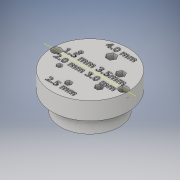
# Autodesk Inventor part: AllenKeyHolder
Saved by Autodesk Inventor 2019.1 (Build 231200000, 200)
## iProperties
Created: 2018-08-31
Part Number: AllenKeyHolder
Material: Generic
Document SubType Name: Modeling
Designer: steele
Density: 1 g/cm^3
Appearance: Default
Author: steele
Autodesk Inventor part; units mm, degrees
(part 1 of 2)
ref_plane "YZ Plane" through (0, 0, 0) normal (1, 0, 0) x (0, 1, 0)
ref_plane "XZ Plane" through (0, 0, 0) normal (0, 1, 0) x (-1, 0, 0)
ref_plane "XY Plane" through (0, 0, 0) normal (0, 0, 1) x (1, 0, 0)
sketch "Sketch1" plane through (0, 0, 0) normal (0, 1, 0) x (-1, 0, 0)
  circle A0 centre (0, 0) radius 20.574
  dimension "d0" = 41.148
  constraints: 1 centre point, 1 coincident
  measures "d0" diameter of A0
extrude "Extrusion1" add sketch "Sketch1" against normal blind 9.525
sketch "Sketch2" plane through (0, -9.525, 0) normal (0, -1, 0) x (1, 0, 0)
  circle A0 centre (0, 0) radius 15.875
  dimension "d3" = 31.75
  constraints: 1 centre point, 1 coincident
  measures "d3" diameter of A0
extrude "Extrusion2" add sketch "Sketch2" along normal blind 9.525
sketch "Sketch4" plane through (0, 0, 0) normal (0, 1, 0) x (1, 0, 0)
  circle A0 centre (0, 0) radius 20.574 projected
  point P0 (18.2245, 0)
  point P1 (-18.2245, 0)
  dimension "d9" = 18.2245
  dimension "d10" = 18.2245
  measures "d9" distance of point (18.224, 0) A0.centre
  measures "d10" distance of point (0, 0) point (-18.224, 0)
hole "Hole1" at (18.2245, 0, 0) at (-18.2245, 0, 0) direction (0, -1, 0) diameter 3.2766 end through all counterbore diameter 4.6482 counterbore depth 2.8448 clearance for "Socket Head Cap Screw" size "#4" standard "Ansi Unified Screw Threads"
sketch "Sketch5" plane through (0, 0, 0) normal (0, 1, 0) x (1, 0, 0)
  circle A0 centre (0, 0) radius 12.065 construction
  line L0 (2.2282, 12.0593) -> (0.9291, 9.8093)
  line L1 (0.9291, 9.8093) -> (-1.6689, 9.8093)
  line L2 (-1.6689, 9.8093) -> (-2.968, 12.0593)
  line L3 (-2.968, 12.0593) -> (-1.6689, 14.3093)
  line L4 (-1.6689, 14.3093) -> (0.9291, 14.3093)
  line L5 (0.9291, 14.3093) -> (2.2282, 12.0593)
  line L6 (12.5681, 6.35) -> (11.4134, 4.35)
  line L7 (11.4134, 4.35) -> (9.104, 4.35)
  line L8 (9.104, 4.35) -> (7.9493, 6.35)
  line L9 (7.9493, 6.35) -> (9.104, 8.35)
  line L10 (9.104, 8.35) -> (11.4134, 8.35)
  line L11 (11.4134, 8.35) -> (12.5681, 6.35)
  line L12 (-28.8036, 0) -> (28.8036, 0) projected
  line L13 (11.639, -3.9593) -> (12.6494, -5.7093)
  line L14 (12.6494, -5.7093) -> (11.639, -7.4593)
  line L15 (11.639, -7.4593) -> (9.6183, -7.4593)
  line L16 (9.6183, -7.4593) -> (8.6079, -5.7093)
  line L17 (8.6079, -5.7093) -> (9.6183, -3.9593)
  line L18 (9.6183, -3.9593) -> (11.639, -3.9593)
  line L19 (1.2359, -10.5593) -> (2.1019, -12.0593)
  line L20 (2.1019, -12.0593) -> (1.2359, -13.5593)
  line L21 (1.2359, -13.5593) -> (-0.4961, -13.5593)
  line L22 (-0.4961, -13.5593) -> (-1.3622, -12.0593)
  line L23 (-1.3622, -12.0593) -> (-0.4961, -10.5593)
  line L24 (-0.4961, -10.5593) -> (1.2359, -10.5593)
  line L25 (-8.8154, -6.35) -> (-9.5371, -7.6)
  line L26 (-9.5371, -7.6) -> (-10.9804, -7.6)
  line L27 (-10.9804, -7.6) -> (-11.7021, -6.35)
  line L28 (-11.7021, -6.35) -> (-10.9804, -5.1)
  line L29 (-10.9804, -5.1) -> (-9.5371, -5.1)
  line L30 (-9.5371, -5.1) -> (-8.8154, -6.35)
  line L31 (-9.4739, 5.7093) -> (-10.0513, 4.7093)
  line L32 (-10.0513, 4.7093) -> (-11.206, 4.7093)
  line L33 (-11.206, 4.7093) -> (-11.7833, 5.7093)
  line L34 (-11.7833, 5.7093) -> (-11.206, 6.7093)
  line L35 (-11.206, 6.7093) -> (-10.0513, 6.7093)
  line L36 (-10.0513, 6.7093) -> (-9.4739, 5.7093)
  point P0 (-0.3699, 12.0593)
  point P1 (-10.6286, 5.7093)
  point P2 (-10.2587, -6.35)
  point P3 (0.3699, -12.0593)
  point P4 (10.6286, -5.7093)
  point P5 (10.2587, 6.35)
  point P6 (-0.3699, 12.0593)
  point P7 (10.2587, 6.35)
  point P8 (10.6286, -5.7093)
  point P9 (0.3699, -12.0593)
  point P10 (-10.2587, -6.35)
  point P11 (-10.6286, 5.7093)
  dimension "d18" = 24.13
  dimension "d21" = 360
  dimension "d23" = 4.5
  dimension "d24" = 4
  dimension "d25" = 3.5
  dimension "d26" = 3
  dimension "d27" = 2.5
  dimension "d28" = 2
  constraints: 72 end point, 7 coincident, 5 parallel, 88 other
  measures "d23" distance between parallel lines of L1 L4
  measures "d24" distance between parallel lines of L7 L10
  measures "d25" distance between parallel lines of L15 L18
  measures "d26" distance between parallel lines of L21 L24
  measures "d27" distance between parallel lines of L26 L29
  measures "d28" distance between parallel lines of L32 L35
extrude "Extrusion4" cut sketch "Sketch5" against normal through all
sketch "Sketch6" plane through (0, 0, 0) normal (0, 1, 0) x (1, 0, 0)
  line L0 (-12.7271, 15.24) -> (13.8214, 15.24) construction
  circle A0 centre (0, 0) radius 20.574 construction
  line L1 (-11.7818, -16.8665) -> (11.7818, -16.8665) construction
  line L2 (-20.5348, 1.27) -> (20.5348, 1.27) construction
  line L3 (-20.1938, -3.937) -> (20.1938, -3.937) construction
  line L4 (-4.8017, 15.9514) -> (-5.2142, 15.9514)
  line L5 (-5.2142, 15.9514) -> (-5.2142, 15.2326)
  line L6 (-5.2142, 15.2326) -> (-5.9527, 15.2326)
  line L7 (-5.9527, 15.2326) -> (-5.9527, 15.9514)
  line L8 (-5.9527, 15.9514) -> (-7.2964, 15.9514)
  line L9 (-7.2964, 15.9514) -> (-7.2964, 16.5195)
  line L10 (-7.2964, 16.5195) -> (-5.9774, 18.288)
  line L11 (-5.9774, 18.288) -> (-5.2142, 18.288)
  line L12 (-5.2142, 18.288) -> (-5.2142, 16.4997)
  line L13 (-5.2142, 16.4997) -> (-4.8017, 16.4997)
  line L14 (-4.8017, 16.4997) -> (-4.8017, 15.9514)
  line L15 (-5.9527, 16.4997) -> (-5.9527, 17.5371)
  line L16 (-5.9527, 17.5371) -> (-6.7258, 16.4997)
  line L17 (-6.7258, 16.4997) -> (-5.9527, 16.4997)
  line L18 (-3.7025, 15.24) -> (-4.4262, 15.24)
  line L19 (-4.4262, 15.24) -> (-4.4262, 16.0452)
  line L20 (-4.4262, 16.0452) -> (-3.7025, 16.0452)
  line L21 (-3.7025, 16.0452) -> (-3.7025, 15.24)
  spline S0 degree 2 poles (-0.899, 16.764) (-0.899, 16.3688) (-1.025, 15.776) (-1.1658, 15.5759) knots 0 0 0 1 2 2 2
  spline S1 degree 2 poles (-1.1658, 15.5759) (-1.3041, 15.3783) (-1.7512, 15.1758) (-2.0723, 15.1758) knots 0 0 0 1 2 2 2
  spline S2 degree 2 poles (-2.0723, 15.1758) (-2.3959, 15.1758) (-2.8405, 15.3783) (-2.9813, 15.5809) knots 0 0 0 1 2 2 2
  spline S3 degree 2 poles (-2.9813, 15.5809) (-3.1221, 15.7809) (-3.248, 16.3688) (-3.248, 16.764) knots 0 0 0 1 2 2 2
  spline S4 degree 2 poles (-3.248, 16.764) (-3.248, 17.1691) (-3.1221, 17.7421) (-2.9788, 17.9496) knots 0 0 0 1 2 2 2
  spline S5 degree 2 poles (-2.9788, 17.9496) (-2.8355, 18.1521) (-2.3835, 18.3498) (-2.0723, 18.3498) knots 0 0 0 1 2 2 2
  spline S6 degree 2 poles (-2.0723, 18.3498) (-1.7438, 18.3498) (-1.3041, 18.1423) (-1.1633, 17.9373) knots 0 0 0 1 2 2 2
  spline S7 degree 2 poles (-1.1633, 17.9373) (-1.025, 17.7372) (-0.899, 17.1469) (-0.899, 16.764) knots 0 0 0 1 2 2 2
  spline S8 degree 2 poles (-1.6672, 16.764) (-1.6672, 17.3296) (-1.8525, 17.7866) (-2.0723, 17.7866) knots 0 0 0 1 2 2 2
  spline S9 degree 2 poles (-2.0723, 17.7866) (-2.2921, 17.7866) (-2.4798, 17.3296) (-2.4798, 16.7615) knots 0 0 0 1 2 2 2
  spline S10 degree 2 poles (-2.4798, 16.7615) (-2.4798, 16.2033) (-2.2921, 15.7389) (-2.0723, 15.7389) knots 0 0 0 1 2 2 2
  spline S11 degree 2 poles (-2.0723, 15.7389) (-1.8549, 15.7389) (-1.6672, 16.2033) (-1.6672, 16.764) knots 0 0 0 1 2 2 2
  line L22 (3.5075, 15.24) -> (3.5075, 16.3886)
  spline S12 degree 2 poles (3.5075, 16.3886) (3.5075, 16.559) (3.4951, 16.7912) (3.4655, 16.8653) knots 0 0 0 1 2 2 2
  spline S13 degree 2 poles (3.4655, 16.8653) (3.4334, 16.9394) (3.3049, 17.0061) (3.1888, 17.0061) knots 0 0 0 1 2 2 2
  spline S14 degree 2 poles (3.1888, 17.0061) (3.1073, 17.0061) (2.9492, 16.9344) (2.8554, 16.8677) knots 0 0 0 1 2 2 2
  line L23 (2.8554, 16.8677) -> (2.8554, 15.24)
  line L24 (2.8554, 15.24) -> (2.1341, 15.24)
  line L25 (2.1341, 15.24) -> (2.1341, 16.3886)
  spline S15 degree 2 poles (2.1341, 16.3886) (2.1341, 16.5565) (2.1193, 16.7912) (2.0897, 16.8653) knots 0 0 0 1 2 2 2
  spline S16 degree 2 poles (2.0897, 16.8653) (2.0576, 16.9394) (1.9291, 17.0061) (1.813, 17.0061) knots 0 0 0 1 2 2 2
  spline S17 degree 2 poles (1.813, 17.0061) (1.7266, 17.0061) (1.5562, 16.9246) (1.4771, 16.8677) knots 0 0 0 1 2 2 2
  line L26 (1.4771, 16.8677) -> (1.4771, 15.24)
  line L27 (1.4771, 15.24) -> (0.7608, 15.24)
  line L28 (0.7608, 15.24) -> (0.7608, 17.5396)
  line L29 (0.7608, 17.5396) -> (1.4771, 17.5396)
  line L30 (1.4771, 17.5396) -> (1.4771, 17.2852)
  spline S18 degree 2 poles (1.4771, 17.2852) (1.6525, 17.4334) (1.9662, 17.6013) (2.1613, 17.6013) knots 0 0 0 1 2 2 2
  spline S19 degree 2 poles (2.1613, 17.6013) (2.3713, 17.6013) (2.6924, 17.4013) (2.7763, 17.2012) knots 0 0 0 1 2 2 2
  spline S20 degree 2 poles (2.7763, 17.2012) (2.9814, 17.3939) (3.3469, 17.6013) (3.5346, 17.6013) knots 0 0 0 1 2 2 2
  spline S21 degree 2 poles (3.5346, 17.6013) (3.6952, 17.6013) (3.9496, 17.5001) (4.0361, 17.3963) knots 0 0 0 1 2 2 2
  spline S22 degree 2 poles (4.0361, 17.3963) (4.1324, 17.2852) (4.2287, 16.9814) (4.2287, 16.7368) knots 0 0 0 1 2 2 2
  line L31 (4.2287, 16.7368) -> (4.2287, 15.24)
  line L32 (4.2287, 15.24) -> (3.5075, 15.24)
  line L33 (7.504, 15.24) -> (7.504, 16.3886)
  spline S23 degree 2 poles (7.504, 16.3886) (7.504, 16.559) (7.4916, 16.7912) (7.462, 16.8653) knots 0 0 0 1 2 2 2
  spline S24 degree 2 poles (7.462, 16.8653) (7.4299, 16.9394) (7.3014, 17.0061) (7.1853, 17.0061) knots 0 0 0 1 2 2 2
  spline S25 degree 2 poles (7.1853, 17.0061) (7.1038, 17.0061) (6.9457, 16.9344) (6.8519, 16.8677) knots 0 0 0 1 2 2 2
  line L34 (6.8519, 16.8677) -> (6.8519, 15.24)
  line L35 (6.8519, 15.24) -> (6.1306, 15.24)
  line L36 (6.1306, 15.24) -> (6.1306, 16.3886)
  spline S26 degree 2 poles (6.1306, 16.3886) (6.1306, 16.5565) (6.1158, 16.7912) (6.0862, 16.8653) knots 0 0 0 1 2 2 2
  spline S27 degree 2 poles (6.0862, 16.8653) (6.0541, 16.9394) (5.9256, 17.0061) (5.8095, 17.0061) knots 0 0 0 1 2 2 2
  spline S28 degree 2 poles (5.8095, 17.0061) (5.7231, 17.0061) (5.5526, 16.9246) (5.4736, 16.8677) knots 0 0 0 1 2 2 2
  line L37 (5.4736, 16.8677) -> (5.4736, 15.24)
  line L38 (5.4736, 15.24) -> (4.7573, 15.24)
  line L39 (4.7573, 15.24) -> (4.7573, 17.5396)
  line L40 (4.7573, 17.5396) -> (5.4736, 17.5396)
  line L41 (5.4736, 17.5396) -> (5.4736, 17.2852)
  spline S29 degree 2 poles (5.4736, 17.2852) (5.649, 17.4334) (5.9627, 17.6013) (6.1578, 17.6013) knots 0 0 0 1 2 2 2
  spline S30 degree 2 poles (6.1578, 17.6013) (6.3678, 17.6013) (6.6889, 17.4013) (6.7728, 17.2012) knots 0 0 0 1 2 2 2
  spline S31 degree 2 poles (6.7728, 17.2012) (6.9778, 17.3939) (7.3434, 17.6013) (7.5311, 17.6013) knots 0 0 0 1 2 2 2
  spline S32 degree 2 poles (7.5311, 17.6013) (7.6917, 17.6013) (7.9461, 17.5001) (8.0325, 17.3963) knots 0 0 0 1 2 2 2
  spline S33 degree 2 poles (8.0325, 17.3963) (8.1289, 17.2852) (8.2252, 16.9814) (8.2252, 16.7368) knots 0 0 0 1 2 2 2
  line L42 (8.2252, 16.7368) -> (8.2252, 15.24)
  line L43 (8.2252, 15.24) -> (7.504, 15.24)
  line L44 (-14.0173, 1.27) -> (-16.1143, 1.27)
  line L45 (-16.1143, 1.27) -> (-16.1143, 1.8232)
  line L46 (-16.1143, 1.8232) -> (-15.4453, 1.8232)
  line L47 (-15.4453, 1.8232) -> (-15.4453, 3.5033)
  line L48 (-15.4453, 3.5033) -> (-16.1143, 3.5033)
  line L49 (-16.1143, 3.5033) -> (-16.1143, 4.0205)
  spline S34 degree 2 poles (-16.1143, 4.0205) (-15.9676, 4.0205) (-15.6769, 4.0591) (-15.5894, 4.1002) knots 0 0 0 1 2 2 2
  spline S35 degree 2 poles (-15.5894, 4.1002) (-15.4891, 4.1517) (-15.3759, 4.3241) (-15.3656, 4.4527) knots 0 0 0 1 2 2 2
  line L50 (-15.3656, 4.4527) -> (-14.6709, 4.4527)
  line L51 (-14.6709, 4.4527) -> (-14.6709, 1.8232)
  line L52 (-14.6709, 1.8232) -> (-14.0173, 1.8232)
  line L53 (-14.0173, 1.8232) -> (-14.0173, 1.27)
  line L54 (-12.6923, 1.27) -> (-13.4462, 1.27)
  line L55 (-13.4462, 1.27) -> (-13.4462, 2.1088)
  line L56 (-13.4462, 2.1088) -> (-12.6923, 2.1088)
  line L57 (-12.6923, 2.1088) -> (-12.6923, 1.27)
  spline S36 degree 2 poles (-9.8029, 2.3455) (-9.8029, 2.0959) (-9.9727, 1.674) (-10.1399, 1.5221) knots 0 0 0 1 2 2 2
  spline S37 degree 2 poles (-10.1399, 1.5221) (-10.3072, 1.3703) (-10.7652, 1.2031) (-11.0996, 1.2031) knots 0 0 0 1 2 2 2
  spline S38 degree 2 poles (-11.0996, 1.2031) (-11.4547, 1.2057) (-11.9641, 1.3215) (-12.1314, 1.3961) knots 0 0 0 1 2 2 2
  line L58 (-12.1314, 1.3961) -> (-12.1314, 2.0882)
  line L59 (-12.1314, 2.0882) -> (-12.0593, 2.0882)
  spline S39 degree 2 poles (-12.0593, 2.0882) (-11.9976, 2.0547) (-11.8484, 1.9673) (-11.7274, 1.921) knots 0 0 0 1 2 2 2
  spline S40 degree 2 poles (-11.7274, 1.921) (-11.6142, 1.8772) (-11.3801, 1.818) (-11.2386, 1.818) knots 0 0 0 1 2 2 2
  spline S41 degree 2 poles (-11.2386, 1.818) (-11.1151, 1.818) (-10.8269, 1.8798) (-10.7394, 1.9621) knots 0 0 0 1 2 2 2
  spline S42 degree 2 poles (-10.7394, 1.9621) (-10.6751, 2.0264) (-10.6031, 2.1834) (-10.6031, 2.3146) knots 0 0 0 1 2 2 2
  spline S43 degree 2 poles (-10.6031, 2.3146) (-10.6031, 2.4278) (-10.6957, 2.5873) (-10.7703, 2.6362) knots 0 0 0 1 2 2 2
  spline S44 degree 2 poles (-10.7703, 2.6362) (-10.8784, 2.7083) (-11.1871, 2.7494) (-11.2978, 2.7494) knots 0 0 0 1 2 2 2
  spline S45 degree 2 poles (-11.2978, 2.7494) (-11.4727, 2.7494) (-11.8046, 2.6928) (-11.9255, 2.662) knots 0 0 0 1 2 2 2
  line L60 (-11.9255, 2.662) -> (-11.995, 2.662)
  line L61 (-11.995, 2.662) -> (-11.995, 4.445)
  line L62 (-11.995, 4.445) -> (-9.8904, 4.445)
  line L63 (-9.8904, 4.445) -> (-9.8904, 3.8455)
  line L64 (-9.8904, 3.8455) -> (-11.2411, 3.8455)
  line L65 (-11.2411, 3.8455) -> (-11.2411, 3.3181)
  spline S46 degree 2 poles (-11.2411, 3.3181) (-11.1768, 3.3232) (-10.9993, 3.3283) (-10.9504, 3.3283) knots 0 0 0 1 2 2 2
  spline S47 degree 2 poles (-10.9504, 3.3283) (-10.7214, 3.3283) (-10.3355, 3.2357) (-10.1837, 3.1405) knots 0 0 0 1 2 2 2
  spline S48 degree 2 poles (-10.1837, 3.1405) (-10.0036, 3.0222) (-9.8029, 2.6285) (-9.8029, 2.3455) knots 0 0 0 1 2 2 2
  line L66 (-5.1819, 1.27) -> (-5.1819, 2.4664)
  spline S49 degree 2 poles (-5.1819, 2.4664) (-5.1819, 2.6439) (-5.1948, 2.8858) (-5.2256, 2.963) knots 0 0 0 1 2 2 2
  spline S50 degree 2 poles (-5.2256, 2.963) (-5.2591, 3.0402) (-5.3929, 3.1096) (-5.5138, 3.1096) knots 0 0 0 1 2 2 2
  spline S51 degree 2 poles (-5.5138, 3.1096) (-5.5987, 3.1096) (-5.7634, 3.035) (-5.8611, 2.9656) knots 0 0 0 1 2 2 2
  line L67 (-5.8611, 2.9656) -> (-5.8611, 1.27)
  line L68 (-5.8611, 1.27) -> (-6.6124, 1.27)
  line L69 (-6.6124, 1.27) -> (-6.6124, 2.4664)
  spline S52 degree 2 poles (-6.6124, 2.4664) (-6.6124, 2.6414) (-6.6279, 2.8858) (-6.6588, 2.963) knots 0 0 0 1 2 2 2
  spline S53 degree 2 poles (-6.6588, 2.963) (-6.6922, 3.0402) (-6.826, 3.1096) (-6.9469, 3.1096) knots 0 0 0 1 2 2 2
  spline S54 degree 2 poles (-6.9469, 3.1096) (-7.037, 3.1096) (-7.2145, 3.0247) (-7.2968, 2.9656) knots 0 0 0 1 2 2 2
  line L70 (-7.2968, 2.9656) -> (-7.2968, 1.27)
  line L71 (-7.2968, 1.27) -> (-8.043, 1.27)
  line L72 (-8.043, 1.27) -> (-8.043, 3.6654)
  line L73 (-8.043, 3.6654) -> (-7.2968, 3.6654)
  line L74 (-7.2968, 3.6654) -> (-7.2968, 3.4004)
  spline S55 degree 2 poles (-7.2968, 3.4004) (-7.1142, 3.5548) (-6.7874, 3.7297) (-6.5841, 3.7297) knots 0 0 0 1 2 2 2
  spline S56 degree 2 poles (-6.5841, 3.7297) (-6.3654, 3.7297) (-6.031, 3.5213) (-5.9435, 3.3129) knots 0 0 0 1 2 2 2
  spline S57 degree 2 poles (-5.9435, 3.3129) (-5.7299, 3.5136) (-5.3491, 3.7297) (-5.1536, 3.7297) knots 0 0 0 1 2 2 2
  spline S58 degree 2 poles (-5.1536, 3.7297) (-4.9863, 3.7297) (-4.7213, 3.6242) (-4.6313, 3.5162) knots 0 0 0 1 2 2 2
  spline S59 degree 2 poles (-4.6313, 3.5162) (-4.5309, 3.4004) (-4.4306, 3.0839) (-4.4306, 2.8292) knots 0 0 0 1 2 2 2
  line L75 (-4.4306, 2.8292) -> (-4.4306, 1.27)
  line L76 (-4.4306, 1.27) -> (-5.1819, 1.27)
  line L77 (-1.0189, 1.27) -> (-1.0189, 2.4664)
  spline S60 degree 2 poles (-1.0189, 2.4664) (-1.0189, 2.6439) (-1.0317, 2.8858) (-1.0626, 2.963) knots 0 0 0 1 2 2 2
  spline S61 degree 2 poles (-1.0626, 2.963) (-1.0961, 3.0402) (-1.2299, 3.1096) (-1.3508, 3.1096) knots 0 0 0 1 2 2 2
  spline S62 degree 2 poles (-1.3508, 3.1096) (-1.4357, 3.1096) (-1.6004, 3.035) (-1.6981, 2.9656) knots 0 0 0 1 2 2 2
  line L78 (-1.6981, 2.9656) -> (-1.6981, 1.27)
  line L79 (-1.6981, 1.27) -> (-2.4494, 1.27)
  line L80 (-2.4494, 1.27) -> (-2.4494, 2.4664)
  spline S63 degree 2 poles (-2.4494, 2.4664) (-2.4494, 2.6414) (-2.4649, 2.8858) (-2.4957, 2.963) knots 0 0 0 1 2 2 2
  spline S64 degree 2 poles (-2.4957, 2.963) (-2.5292, 3.0402) (-2.663, 3.1096) (-2.7839, 3.1096) knots 0 0 0 1 2 2 2
  spline S65 degree 2 poles (-2.7839, 3.1096) (-2.874, 3.1096) (-3.0515, 3.0247) (-3.1338, 2.9656) knots 0 0 0 1 2 2 2
  line L81 (-3.1338, 2.9656) -> (-3.1338, 1.27)
  line L82 (-3.1338, 1.27) -> (-3.88, 1.27)
  line L83 (-3.88, 1.27) -> (-3.88, 3.6654)
  line L84 (-3.88, 3.6654) -> (-3.1338, 3.6654)
  line L85 (-3.1338, 3.6654) -> (-3.1338, 3.4004)
  spline S66 degree 2 poles (-3.1338, 3.4004) (-2.9512, 3.5548) (-2.6244, 3.7297) (-2.4211, 3.7297) knots 0 0 0 1 2 2 2
  spline S67 degree 2 poles (-2.4211, 3.7297) (-2.2024, 3.7297) (-1.868, 3.5213) (-1.7805, 3.3129) knots 0 0 0 1 2 2 2
  spline S68 degree 2 poles (-1.7805, 3.3129) (-1.5669, 3.5136) (-1.1861, 3.7297) (-0.9906, 3.7297) knots 0 0 0 1 2 2 2
  spline S69 degree 2 poles (-0.9906, 3.7297) (-0.8233, 3.7297) (-0.5583, 3.6242) (-0.4683, 3.5162) knots 0 0 0 1 2 2 2
  spline S70 degree 2 poles (-0.4683, 3.5162) (-0.3679, 3.4004) (-0.2676, 3.0839) (-0.2676, 2.8292) knots 0 0 0 1 2 2 2
  line L86 (-0.2676, 2.8292) -> (-0.2676, 1.27)
  line L87 (-0.2676, 1.27) -> (-1.0189, 1.27)
  spline S71 degree 2 poles (3.8543, 2.2323) (3.8543, 1.9981) (3.6819, 1.6148) (3.5146, 1.481) knots 0 0 0 1 2 2 2
  spline S72 degree 2 poles (3.5146, 1.481) (3.3474, 1.3472) (2.892, 1.2031) (2.5652, 1.2031) knots 0 0 0 1 2 2 2
  spline S73 degree 2 poles (2.5652, 1.2031) (2.1947, 1.2031) (1.6647, 1.3266) (1.4974, 1.4038) knots 0 0 0 1 2 2 2
  line L88 (1.4974, 1.4038) -> (1.4974, 2.0933)
  line L89 (1.4974, 2.0933) -> (1.5746, 2.0933)
  spline S74 degree 2 poles (1.5746, 2.0933) (1.7496, 1.9827) (2.2204, 1.818) (2.416, 1.818) knots 0 0 0 1 2 2 2
  spline S75 degree 2 poles (2.416, 1.818) (2.5318, 1.818) (2.8019, 1.8592) (2.8945, 1.9261) knots 0 0 0 1 2 2 2
  spline S76 degree 2 poles (2.8945, 1.9261) (2.9666, 1.9801) (3.0541, 2.1371) (3.0541, 2.2786) knots 0 0 0 1 2 2 2
  spline S77 degree 2 poles (3.0541, 2.2786) (3.0541, 2.4201) (2.9306, 2.5719) (2.8277, 2.6079) knots 0 0 0 1 2 2 2
  spline S78 degree 2 poles (2.8277, 2.6079) (2.7247, 2.6439) (2.4391, 2.6517) (2.3285, 2.6517) knots 0 0 0 1 2 2 2
  line L90 (2.3285, 2.6517) -> (2.1921, 2.6517)
  line L91 (2.1921, 2.6517) -> (2.1921, 3.21)
  line L92 (2.1921, 3.21) -> (2.3182, 3.21)
  spline S79 degree 2 poles (2.3182, 3.21) (2.4623, 3.21) (2.7067, 3.2357) (2.7916, 3.2743) knots 0 0 0 1 2 2 2
  spline S80 degree 2 poles (2.7916, 3.2743) (2.8765, 3.3155) (2.9717, 3.4596) (2.9717, 3.5831) knots 0 0 0 1 2 2 2
  spline S81 degree 2 poles (2.9717, 3.5831) (2.9717, 3.6808) (2.8817, 3.8018) (2.8174, 3.8352) knots 0 0 0 1 2 2 2
  spline S82 degree 2 poles (2.8174, 3.8352) (2.7402, 3.8738) (2.5343, 3.8995) (2.4623, 3.8995) knots 0 0 0 1 2 2 2
  spline S83 degree 2 poles (2.4623, 3.8995) (2.3465, 3.8995) (2.1021, 3.8455) (1.9889, 3.8018) knots 0 0 0 1 2 2 2
  spline S84 degree 2 poles (1.9889, 3.8018) (1.8988, 3.7683) (1.7033, 3.6603) (1.657, 3.632) knots 0 0 0 1 2 2 2
  line L93 (1.657, 3.632) -> (1.5901, 3.632)
  line L94 (1.5901, 3.632) -> (1.5901, 4.3112)
  spline S85 degree 2 poles (1.5901, 4.3112) (1.7547, 4.3807) (2.3105, 4.5119) (2.6012, 4.5119) knots 0 0 0 1 2 2 2
  spline S86 degree 2 poles (2.6012, 4.5119) (2.8843, 4.5119) (3.3011, 4.4141) (3.4477, 4.3189) knots 0 0 0 1 2 2 2
  spline S87 degree 2 poles (3.4477, 4.3189) (3.6098, 4.2186) (3.7719, 3.9098) (3.7719, 3.7169) knots 0 0 0 1 2 2 2
  spline S88 degree 2 poles (3.7719, 3.7169) (3.7719, 3.4441) (3.458, 3.0376) (3.2007, 2.9784) knots 0 0 0 1 2 2 2
  line L95 (3.2007, 2.9784) -> (3.2007, 2.9476)
  spline S89 degree 2 poles (3.2007, 2.9476) (3.3139, 2.9321) (3.5301, 2.8498) (3.633, 2.7572) knots 0 0 0 1 2 2 2
  spline S90 degree 2 poles (3.633, 2.7572) (3.7282, 2.6748) (3.8543, 2.4124) (3.8543, 2.2323) knots 0 0 0 1 2 2 2
  line L96 (5.1176, 1.27) -> (4.3637, 1.27)
  line L97 (4.3637, 1.27) -> (4.3637, 2.1088)
  line L98 (4.3637, 2.1088) -> (5.1176, 2.1088)
  line L99 (5.1176, 2.1088) -> (5.1176, 1.27)
  spline S91 degree 2 poles (8.007, 2.3455) (8.007, 2.0959) (7.8372, 1.674) (7.6699, 1.5221) knots 0 0 0 1 2 2 2
  spline S92 degree 2 poles (7.6699, 1.5221) (7.5027, 1.3703) (7.0447, 1.2031) (6.7102, 1.2031) knots 0 0 0 1 2 2 2
  spline S93 degree 2 poles (6.7102, 1.2031) (6.3551, 1.2057) (5.8457, 1.3215) (5.6785, 1.3961) knots 0 0 0 1 2 2 2
  line L100 (5.6785, 1.3961) -> (5.6785, 2.0882)
  line L101 (5.6785, 2.0882) -> (5.7505, 2.0882)
  spline S94 degree 2 poles (5.7505, 2.0882) (5.8123, 2.0547) (5.9615, 1.9673) (6.0824, 1.921) knots 0 0 0 1 2 2 2
  spline S95 degree 2 poles (6.0824, 1.921) (6.1956, 1.8772) (6.4298, 1.818) (6.5713, 1.818) knots 0 0 0 1 2 2 2
  spline S96 degree 2 poles (6.5713, 1.818) (6.6948, 1.818) (6.9829, 1.8798) (7.0704, 1.9621) knots 0 0 0 1 2 2 2
  spline S97 degree 2 poles (7.0704, 1.9621) (7.1347, 2.0264) (7.2068, 2.1834) (7.2068, 2.3146) knots 0 0 0 1 2 2 2
  spline S98 degree 2 poles (7.2068, 2.3146) (7.2068, 2.4278) (7.1142, 2.5873) (7.0395, 2.6362) knots 0 0 0 1 2 2 2
  spline S99 degree 2 poles (7.0395, 2.6362) (6.9315, 2.7083) (6.6227, 2.7494) (6.5121, 2.7494) knots 0 0 0 1 2 2 2
  spline S100 degree 2 poles (6.5121, 2.7494) (6.3371, 2.7494) (6.0052, 2.6928) (5.8843, 2.662) knots 0 0 0 1 2 2 2
  line L102 (5.8843, 2.662) -> (5.8148, 2.662)
  line L103 (5.8148, 2.662) -> (5.8148, 4.445)
  line L104 (5.8148, 4.445) -> (7.9195, 4.445)
  line L105 (7.9195, 4.445) -> (7.9195, 3.8455)
  line L106 (7.9195, 3.8455) -> (6.5687, 3.8455)
  line L107 (6.5687, 3.8455) -> (6.5687, 3.3181)
  spline S101 degree 2 poles (6.5687, 3.3181) (6.633, 3.3232) (6.8106, 3.3283) (6.8594, 3.3283) knots 0 0 0 1 2 2 2
  spline S102 degree 2 poles (6.8594, 3.3283) (7.0884, 3.3283) (7.4744, 3.2357) (7.6262, 3.1405) knots 0 0 0 1 2 2 2
  spline S103 degree 2 poles (7.6262, 3.1405) (7.8063, 3.0222) (8.007, 2.6285) (8.007, 2.3455) knots 0 0 0 1 2 2 2
  line L108 (11.3492, 1.27) -> (11.3492, 2.4664)
  spline S104 degree 2 poles (11.3492, 2.4664) (11.3492, 2.6439) (11.3363, 2.8858) (11.3055, 2.963) knots 0 0 0 1 2 2 2
  spline S105 degree 2 poles (11.3055, 2.963) (11.272, 3.0402) (11.1382, 3.1096) (11.0173, 3.1096) knots 0 0 0 1 2 2 2
  spline S106 degree 2 poles (11.0173, 3.1096) (10.9324, 3.1096) (10.7677, 3.035) (10.67, 2.9656) knots 0 0 0 1 2 2 2
  line L109 (10.67, 2.9656) -> (10.67, 1.27)
  line L110 (10.67, 1.27) -> (9.9187, 1.27)
  line L111 (9.9187, 1.27) -> (9.9187, 2.4664)
  spline S107 degree 2 poles (9.9187, 2.4664) (9.9187, 2.6414) (9.9032, 2.8858) (9.8723, 2.963) knots 0 0 0 1 2 2 2
  spline S108 degree 2 poles (9.8723, 2.963) (9.8389, 3.0402) (9.7051, 3.1096) (9.5842, 3.1096) knots 0 0 0 1 2 2 2
  spline S109 degree 2 poles (9.5842, 3.1096) (9.4941, 3.1096) (9.3166, 3.0247) (9.2343, 2.9656) knots 0 0 0 1 2 2 2
  line L112 (9.2343, 2.9656) -> (9.2343, 1.27)
  line L113 (9.2343, 1.27) -> (8.4881, 1.27)
  line L114 (8.4881, 1.27) -> (8.4881, 3.6654)
  line L115 (8.4881, 3.6654) -> (9.2343, 3.6654)
  line L116 (9.2343, 3.6654) -> (9.2343, 3.4004)
  spline S110 degree 2 poles (9.2343, 3.4004) (9.4169, 3.5548) (9.7437, 3.7297) (9.947, 3.7297) knots 0 0 0 1 2 2 2
  spline S111 degree 2 poles (9.947, 3.7297) (10.1657, 3.7297) (10.5001, 3.5213) (10.5876, 3.3129) knots 0 0 0 1 2 2 2
  spline S112 degree 2 poles (10.5876, 3.3129) (10.8012, 3.5136) (11.182, 3.7297) (11.3775, 3.7297) knots 0 0 0 1 2 2 2
  spline S113 degree 2 poles (11.3775, 3.7297) (11.5448, 3.7297) (11.8098, 3.6242) (11.8998, 3.5162) knots 0 0 0 1 2 2 2
  spline S114 degree 2 poles (11.8998, 3.5162) (12.0002, 3.4004) (12.1005, 3.0839) (12.1005, 2.8292) knots 0 0 0 1 2 2 2
  line L117 (12.1005, 2.8292) -> (12.1005, 1.27)
  line L118 (12.1005, 1.27) -> (11.3492, 1.27)
  line L119 (15.5122, 1.27) -> (15.5122, 2.4664)
  spline S115 degree 2 poles (15.5122, 2.4664) (15.5122, 2.6439) (15.4994, 2.8858) (15.4685, 2.963) knots 0 0 0 1 2 2 2
  spline S116 degree 2 poles (15.4685, 2.963) (15.435, 3.0402) (15.3012, 3.1096) (15.1803, 3.1096) knots 0 0 0 1 2 2 2
  spline S117 degree 2 poles (15.1803, 3.1096) (15.0954, 3.1096) (14.9307, 3.035) (14.833, 2.9656) knots 0 0 0 1 2 2 2
  line L120 (14.833, 2.9656) -> (14.833, 1.27)
  line L121 (14.833, 1.27) -> (14.0817, 1.27)
  line L122 (14.0817, 1.27) -> (14.0817, 2.4664)
  spline S118 degree 2 poles (14.0817, 2.4664) (14.0817, 2.6414) (14.0662, 2.8858) (14.0354, 2.963) knots 0 0 0 1 2 2 2
  spline S119 degree 2 poles (14.0354, 2.963) (14.0019, 3.0402) (13.8681, 3.1096) (13.7472, 3.1096) knots 0 0 0 1 2 2 2
  spline S120 degree 2 poles (13.7472, 3.1096) (13.6571, 3.1096) (13.4796, 3.0247) (13.3973, 2.9656) knots 0 0 0 1 2 2 2
  line L123 (13.3973, 2.9656) -> (13.3973, 1.27)
  line L124 (13.3973, 1.27) -> (12.6511, 1.27)
  line L125 (12.6511, 1.27) -> (12.6511, 3.6654)
  line L126 (12.6511, 3.6654) -> (13.3973, 3.6654)
  line L127 (13.3973, 3.6654) -> (13.3973, 3.4004)
  spline S121 degree 2 poles (13.3973, 3.4004) (13.5799, 3.5548) (13.9067, 3.7297) (14.11, 3.7297) knots 0 0 0 1 2 2 2
  spline S122 degree 2 poles (14.11, 3.7297) (14.3287, 3.7297) (14.6631, 3.5213) (14.7506, 3.3129) knots 0 0 0 1 2 2 2
  spline S123 degree 2 poles (14.7506, 3.3129) (14.9642, 3.5136) (15.345, 3.7297) (15.5405, 3.7297) knots 0 0 0 1 2 2 2
  spline S124 degree 2 poles (15.5405, 3.7297) (15.7078, 3.7297) (15.9728, 3.6242) (16.0628, 3.5162) knots 0 0 0 1 2 2 2
  spline S125 degree 2 poles (16.0628, 3.5162) (16.1632, 3.4004) (16.2635, 3.0839) (16.2635, 2.8292) knots 0 0 0 1 2 2 2
  line L128 (16.2635, 2.8292) -> (16.2635, 1.27)
  line L129 (16.2635, 1.27) -> (15.5122, 1.27)
  line L130 (-13.9346, -3.937) -> (-16.1749, -3.937)
  line L131 (-16.1749, -3.937) -> (-16.1749, -3.4405)
  spline S126 degree 2 poles (-16.1749, -3.4405) (-15.8908, -3.2133) (-15.4364, -2.8131) (-15.2659, -2.6328) knots 0 0 0 1 2 2 2
  spline S127 degree 2 poles (-15.2659, -2.6328) (-15.0412, -2.3982) (-14.8411, -2.04) (-14.8411, -1.8523) knots 0 0 0 1 2 2 2
  spline S128 degree 2 poles (-14.8411, -1.8523) (-14.8411, -1.6399) (-15.0955, -1.4126) (-15.3227, -1.4126) knots 0 0 0 1 2 2 2
  spline S129 degree 2 poles (-15.3227, -1.4126) (-15.4388, -1.4126) (-15.6463, -1.4695) (-15.7525, -1.5139) knots 0 0 0 1 2 2 2
  spline S130 degree 2 poles (-15.7525, -1.5139) (-15.8563, -1.5608) (-16.0045, -1.6596) (-16.0415, -1.6843) knots 0 0 0 1 2 2 2
  line L132 (-16.0415, -1.6843) -> (-16.1008, -1.6843)
  line L133 (-16.1008, -1.6843) -> (-16.1008, -1.0199)
  spline S131 degree 2 poles (-16.1008, -1.0199) (-15.9724, -0.9582) (-15.424, -0.8297) (-15.1696, -0.8297) knots 0 0 0 1 2 2 2
  spline S132 degree 2 poles (-15.1696, -0.8297) (-14.6262, -0.8297) (-14.068, -1.3138) (-14.068, -1.751) knots 0 0 0 1 2 2 2
  spline S133 degree 2 poles (-14.068, -1.751) (-14.068, -2.0203) (-14.3224, -2.539) (-14.6163, -2.8354) knots 0 0 0 1 2 2 2
  spline S134 degree 2 poles (-14.6163, -2.8354) (-14.8016, -3.0182) (-15.1498, -3.3022) (-15.2264, -3.3615) knots 0 0 0 1 2 2 2
  line L134 (-15.2264, -3.3615) -> (-13.9346, -3.3615)
  line L135 (-13.9346, -3.3615) -> (-13.9346, -3.937)
  line L136 (-12.7984, -3.937) -> (-13.5221, -3.937)
  line L137 (-13.5221, -3.937) -> (-13.5221, -3.1318)
  line L138 (-13.5221, -3.1318) -> (-12.7984, -3.1318)
  line L139 (-12.7984, -3.1318) -> (-12.7984, -3.937)
  spline S135 degree 2 poles (-9.9949, -2.413) (-9.9949, -2.8082) (-10.1209, -3.401) (-10.2617, -3.6011) knots 0 0 0 1 2 2 2
  spline S136 degree 2 poles (-10.2617, -3.6011) (-10.4, -3.7987) (-10.8471, -4.0012) (-11.1682, -4.0012) knots 0 0 0 1 2 2 2
  spline S137 degree 2 poles (-11.1682, -4.0012) (-11.4917, -4.0012) (-11.9364, -3.7987) (-12.0771, -3.5961) knots 0 0 0 1 2 2 2
  spline S138 degree 2 poles (-12.0771, -3.5961) (-12.2179, -3.3961) (-12.3439, -2.8082) (-12.3439, -2.413) knots 0 0 0 1 2 2 2
  spline S139 degree 2 poles (-12.3439, -2.413) (-12.3439, -2.0079) (-12.2179, -1.4349) (-12.0747, -1.2274) knots 0 0 0 1 2 2 2
  spline S140 degree 2 poles (-12.0747, -1.2274) (-11.9314, -1.0249) (-11.4794, -0.8272) (-11.1682, -0.8272) knots 0 0 0 1 2 2 2
  spline S141 degree 2 poles (-11.1682, -0.8272) (-10.8397, -0.8272) (-10.4, -1.0347) (-10.2592, -1.2397) knots 0 0 0 1 2 2 2
  spline S142 degree 2 poles (-10.2592, -1.2397) (-10.1209, -1.4398) (-9.9949, -2.0301) (-9.9949, -2.413) knots 0 0 0 1 2 2 2
  spline S143 degree 2 poles (-10.7631, -2.413) (-10.7631, -1.8474) (-10.9483, -1.3904) (-11.1682, -1.3904) knots 0 0 0 1 2 2 2
  spline S144 degree 2 poles (-11.1682, -1.3904) (-11.388, -1.3904) (-11.5757, -1.8474) (-11.5757, -2.4155) knots 0 0 0 1 2 2 2
  spline S145 degree 2 poles (-11.5757, -2.4155) (-11.5757, -2.9737) (-11.388, -3.4381) (-11.1682, -3.4381) knots 0 0 0 1 2 2 2
  spline S146 degree 2 poles (-11.1682, -3.4381) (-10.9508, -3.4381) (-10.7631, -2.9737) (-10.7631, -2.413) knots 0 0 0 1 2 2 2
  line L140 (-5.5884, -3.937) -> (-5.5884, -2.7884)
  spline S147 degree 2 poles (-5.5884, -2.7884) (-5.5884, -2.618) (-5.6008, -2.3858) (-5.6304, -2.3117) knots 0 0 0 1 2 2 2
  spline S148 degree 2 poles (-5.6304, -2.3117) (-5.6625, -2.2376) (-5.791, -2.1709) (-5.907, -2.1709) knots 0 0 0 1 2 2 2
  spline S149 degree 2 poles (-5.907, -2.1709) (-5.9886, -2.1709) (-6.1466, -2.2426) (-6.2405, -2.3093) knots 0 0 0 1 2 2 2
  line L141 (-6.2405, -2.3093) -> (-6.2405, -3.937)
  line L142 (-6.2405, -3.937) -> (-6.9617, -3.937)
  line L143 (-6.9617, -3.937) -> (-6.9617, -2.7884)
  spline S150 degree 2 poles (-6.9617, -2.7884) (-6.9617, -2.6205) (-6.9766, -2.3858) (-7.0062, -2.3117) knots 0 0 0 1 2 2 2
  spline S151 degree 2 poles (-7.0062, -2.3117) (-7.0383, -2.2376) (-7.1668, -2.1709) (-7.2828, -2.1709) knots 0 0 0 1 2 2 2
  spline S152 degree 2 poles (-7.2828, -2.1709) (-7.3693, -2.1709) (-7.5397, -2.2524) (-7.6188, -2.3093) knots 0 0 0 1 2 2 2
  line L144 (-7.6188, -2.3093) -> (-7.6188, -3.937)
  line L145 (-7.6188, -3.937) -> (-8.3351, -3.937)
  line L146 (-8.3351, -3.937) -> (-8.3351, -1.6374)
  line L147 (-8.3351, -1.6374) -> (-7.6188, -1.6374)
  line L148 (-7.6188, -1.6374) -> (-7.6188, -1.8918)
  spline S153 degree 2 poles (-7.6188, -1.8918) (-7.4434, -1.7436) (-7.1297, -1.5757) (-6.9346, -1.5757) knots 0 0 0 1 2 2 2
  spline S154 degree 2 poles (-6.9346, -1.5757) (-6.7246, -1.5757) (-6.4035, -1.7757) (-6.3195, -1.9758) knots 0 0 0 1 2 2 2
  spline S155 degree 2 poles (-6.3195, -1.9758) (-6.1145, -1.7831) (-5.749, -1.5757) (-5.5612, -1.5757) knots 0 0 0 1 2 2 2
  spline S156 degree 2 poles (-5.5612, -1.5757) (-5.4007, -1.5757) (-5.1463, -1.6769) (-5.0598, -1.7807) knots 0 0 0 1 2 2 2
  spline S157 degree 2 poles (-5.0598, -1.7807) (-4.9635, -1.8918) (-4.8672, -2.1956) (-4.8672, -2.4402) knots 0 0 0 1 2 2 2
  line L149 (-4.8672, -2.4402) -> (-4.8672, -3.937)
  line L150 (-4.8672, -3.937) -> (-5.5884, -3.937)
  line L151 (-1.5919, -3.937) -> (-1.5919, -2.7884)
  spline S158 degree 2 poles (-1.5919, -2.7884) (-1.5919, -2.618) (-1.6043, -2.3858) (-1.6339, -2.3117) knots 0 0 0 1 2 2 2
  spline S159 degree 2 poles (-1.6339, -2.3117) (-1.666, -2.2376) (-1.7945, -2.1709) (-1.9106, -2.1709) knots 0 0 0 1 2 2 2
  spline S160 degree 2 poles (-1.9106, -2.1709) (-1.9921, -2.1709) (-2.1501, -2.2426) (-2.244, -2.3093) knots 0 0 0 1 2 2 2
  line L152 (-2.244, -2.3093) -> (-2.244, -3.937)
  line L153 (-2.244, -3.937) -> (-2.9653, -3.937)
  line L154 (-2.9653, -3.937) -> (-2.9653, -2.7884)
  spline S161 degree 2 poles (-2.9653, -2.7884) (-2.9653, -2.6205) (-2.9801, -2.3858) (-3.0097, -2.3117) knots 0 0 0 1 2 2 2
  spline S162 degree 2 poles (-3.0097, -2.3117) (-3.0418, -2.2376) (-3.1703, -2.1709) (-3.2864, -2.1709) knots 0 0 0 1 2 2 2
  spline S163 degree 2 poles (-3.2864, -2.1709) (-3.3728, -2.1709) (-3.5432, -2.2524) (-3.6223, -2.3093) knots 0 0 0 1 2 2 2
  line L155 (-3.6223, -2.3093) -> (-3.6223, -3.937)
  line L156 (-3.6223, -3.937) -> (-4.3386, -3.937)
  line L157 (-4.3386, -3.937) -> (-4.3386, -1.6374)
  line L158 (-4.3386, -1.6374) -> (-3.6223, -1.6374)
  line L159 (-3.6223, -1.6374) -> (-3.6223, -1.8918)
  spline S164 degree 2 poles (-3.6223, -1.8918) (-3.4469, -1.7436) (-3.1332, -1.5757) (-2.9381, -1.5757) knots 0 0 0 1 2 2 2
  spline S165 degree 2 poles (-2.9381, -1.5757) (-2.7281, -1.5757) (-2.407, -1.7757) (-2.323, -1.9758) knots 0 0 0 1 2 2 2
  spline S166 degree 2 poles (-2.323, -1.9758) (-2.118, -1.7831) (-1.7525, -1.5757) (-1.5648, -1.5757) knots 0 0 0 1 2 2 2
  spline S167 degree 2 poles (-1.5648, -1.5757) (-1.4042, -1.5757) (-1.1498, -1.6769) (-1.0633, -1.7807) knots 0 0 0 1 2 2 2
  spline S168 degree 2 poles (-1.0633, -1.7807) (-0.967, -1.8918) (-0.8707, -2.1956) (-0.8707, -2.4402) knots 0 0 0 1 2 2 2
  line L160 (-0.8707, -2.4402) -> (-0.8707, -3.937)
  line L161 (-0.8707, -3.937) -> (-1.5919, -3.937)
  spline S169 degree 2 poles (3.0863, -3.0132) (3.0863, -3.238) (2.9208, -3.606) (2.7602, -3.7345) knots 0 0 0 1 2 2 2
  spline S170 degree 2 poles (2.7602, -3.7345) (2.5997, -3.8629) (2.1625, -4.0012) (1.8488, -4.0012) knots 0 0 0 1 2 2 2
  spline S171 degree 2 poles (1.8488, -4.0012) (1.4931, -4.0012) (0.9843, -3.8827) (0.8238, -3.8086) knots 0 0 0 1 2 2 2
  line L162 (0.8238, -3.8086) -> (0.8238, -3.1466)
  line L163 (0.8238, -3.1466) -> (0.8979, -3.1466)
  spline S172 degree 2 poles (0.8979, -3.1466) (1.0658, -3.2528) (1.5178, -3.4109) (1.7055, -3.4109) knots 0 0 0 1 2 2 2
  spline S173 degree 2 poles (1.7055, -3.4109) (1.8167, -3.4109) (2.076, -3.3714) (2.165, -3.3071) knots 0 0 0 1 2 2 2
  spline S174 degree 2 poles (2.165, -3.3071) (2.2341, -3.2553) (2.3181, -3.1046) (2.3181, -2.9688) knots 0 0 0 1 2 2 2
  spline S175 degree 2 poles (2.3181, -2.9688) (2.3181, -2.8329) (2.1995, -2.6872) (2.1007, -2.6526) knots 0 0 0 1 2 2 2
  spline S176 degree 2 poles (2.1007, -2.6526) (2.0019, -2.618) (1.7278, -2.6106) (1.6216, -2.6106) knots 0 0 0 1 2 2 2
  line L164 (1.6216, -2.6106) -> (1.4907, -2.6106)
  line L165 (1.4907, -2.6106) -> (1.4907, -2.0746)
  line L166 (1.4907, -2.0746) -> (1.6117, -2.0746)
  spline S177 degree 2 poles (1.6117, -2.0746) (1.75, -2.0746) (1.9847, -2.0499) (2.0662, -2.0129) knots 0 0 0 1 2 2 2
  spline S178 degree 2 poles (2.0662, -2.0129) (2.1477, -1.9733) (2.2391, -1.835) (2.2391, -1.7165) knots 0 0 0 1 2 2 2
  spline S179 degree 2 poles (2.2391, -1.7165) (2.2391, -1.6226) (2.1526, -1.5065) (2.0909, -1.4744) knots 0 0 0 1 2 2 2
  spline S180 degree 2 poles (2.0909, -1.4744) (2.0168, -1.4373) (1.8192, -1.4126) (1.75, -1.4126) knots 0 0 0 1 2 2 2
  spline S181 degree 2 poles (1.75, -1.4126) (1.6389, -1.4126) (1.4042, -1.4645) (1.2955, -1.5065) knots 0 0 0 1 2 2 2
  spline S182 degree 2 poles (1.2955, -1.5065) (1.2091, -1.5386) (1.0214, -1.6424) (0.9769, -1.6695) knots 0 0 0 1 2 2 2
  line L167 (0.9769, -1.6695) -> (0.9127, -1.6695)
  line L168 (0.9127, -1.6695) -> (0.9127, -1.0174)
  spline S183 degree 2 poles (0.9127, -1.0174) (1.0708, -0.9508) (1.6043, -0.8248) (1.8834, -0.8248) knots 0 0 0 1 2 2 2
  spline S184 degree 2 poles (1.8834, -0.8248) (2.1551, -0.8248) (2.5552, -0.9186) (2.696, -1.01) knots 0 0 0 1 2 2 2
  spline S185 degree 2 poles (2.696, -1.01) (2.8516, -1.1064) (3.0072, -1.4028) (3.0072, -1.588) knots 0 0 0 1 2 2 2
  spline S186 degree 2 poles (3.0072, -1.588) (3.0072, -1.8498) (2.7059, -2.2401) (2.4589, -2.2969) knots 0 0 0 1 2 2 2
  line L169 (2.4589, -2.2969) -> (2.4589, -2.3265)
  spline S187 degree 2 poles (2.4589, -2.3265) (2.5676, -2.3414) (2.7751, -2.4204) (2.8739, -2.5093) knots 0 0 0 1 2 2 2
  spline S188 degree 2 poles (2.8739, -2.5093) (2.9653, -2.5884) (3.0863, -2.8403) (3.0863, -3.0132) knots 0 0 0 1 2 2 2
  line L170 (4.2991, -3.937) -> (3.5753, -3.937)
  line L171 (3.5753, -3.937) -> (3.5753, -3.1318)
  line L172 (3.5753, -3.1318) -> (4.2991, -3.1318)
  line L173 (4.2991, -3.1318) -> (4.2991, -3.937)
  spline S189 degree 2 poles (7.1025, -2.413) (7.1025, -2.8082) (6.9766, -3.401) (6.8358, -3.6011) knots 0 0 0 1 2 2 2
  spline S190 degree 2 poles (6.8358, -3.6011) (6.6974, -3.7987) (6.2504, -4.0012) (5.9293, -4.0012) knots 0 0 0 1 2 2 2
  spline S191 degree 2 poles (5.9293, -4.0012) (5.6057, -4.0012) (5.1611, -3.7987) (5.0203, -3.5961) knots 0 0 0 1 2 2 2
  spline S192 degree 2 poles (5.0203, -3.5961) (4.8795, -3.3961) (4.7535, -2.8082) (4.7535, -2.413) knots 0 0 0 1 2 2 2
  spline S193 degree 2 poles (4.7535, -2.413) (4.7535, -2.0079) (4.8795, -1.4349) (5.0228, -1.2274) knots 0 0 0 1 2 2 2
  spline S194 degree 2 poles (5.0228, -1.2274) (5.166, -1.0249) (5.6181, -0.8272) (5.9293, -0.8272) knots 0 0 0 1 2 2 2
  spline S195 degree 2 poles (5.9293, -0.8272) (6.2578, -0.8272) (6.6974, -1.0347) (6.8382, -1.2397) knots 0 0 0 1 2 2 2
  spline S196 degree 2 poles (6.8382, -1.2397) (6.9766, -1.4398) (7.1025, -2.0301) (7.1025, -2.413) knots 0 0 0 1 2 2 2
  spline S197 degree 2 poles (6.3344, -2.413) (6.3344, -1.8474) (6.1491, -1.3904) (5.9293, -1.3904) knots 0 0 0 1 2 2 2
  spline S198 degree 2 poles (5.9293, -1.3904) (5.7094, -1.3904) (5.5217, -1.8474) (5.5217, -2.4155) knots 0 0 0 1 2 2 2
  spline S199 degree 2 poles (5.5217, -2.4155) (5.5217, -2.9737) (5.7094, -3.4381) (5.9293, -3.4381) knots 0 0 0 1 2 2 2
  spline S200 degree 2 poles (5.9293, -3.4381) (6.1466, -3.4381) (6.3344, -2.9737) (6.3344, -2.413) knots 0 0 0 1 2 2 2
  line L174 (11.509, -3.937) -> (11.509, -2.7884)
  spline S201 degree 2 poles (11.509, -2.7884) (11.509, -2.618) (11.4967, -2.3858) (11.4671, -2.3117) knots 0 0 0 1 2 2 2
  spline S202 degree 2 poles (11.4671, -2.3117) (11.4349, -2.2376) (11.3065, -2.1709) (11.1904, -2.1709) knots 0 0 0 1 2 2 2
  spline S203 degree 2 poles (11.1904, -2.1709) (11.1089, -2.1709) (10.9508, -2.2426) (10.857, -2.3093) knots 0 0 0 1 2 2 2
  line L175 (10.857, -2.3093) -> (10.857, -3.937)
  line L176 (10.857, -3.937) -> (10.1357, -3.937)
  line L177 (10.1357, -3.937) -> (10.1357, -2.7884)
  spline S204 degree 2 poles (10.1357, -2.7884) (10.1357, -2.6205) (10.1209, -2.3858) (10.0913, -2.3117) knots 0 0 0 1 2 2 2
  spline S205 degree 2 poles (10.0913, -2.3117) (10.0591, -2.2376) (9.9307, -2.1709) (9.8146, -2.1709) knots 0 0 0 1 2 2 2
  spline S206 degree 2 poles (9.8146, -2.1709) (9.7282, -2.1709) (9.5577, -2.2524) (9.4787, -2.3093) knots 0 0 0 1 2 2 2
  line L178 (9.4787, -2.3093) -> (9.4787, -3.937)
  line L179 (9.4787, -3.937) -> (8.7624, -3.937)
  line L180 (8.7624, -3.937) -> (8.7624, -1.6374)
  line L181 (8.7624, -1.6374) -> (9.4787, -1.6374)
  line L182 (9.4787, -1.6374) -> (9.4787, -1.8918)
  spline S207 degree 2 poles (9.4787, -1.8918) (9.6541, -1.7436) (9.9678, -1.5757) (10.1629, -1.5757) knots 0 0 0 1 2 2 2
  spline S208 degree 2 poles (10.1629, -1.5757) (10.3728, -1.5757) (10.6939, -1.7757) (10.7779, -1.9758) knots 0 0 0 1 2 2 2
  spline S209 degree 2 poles (10.7779, -1.9758) (10.9829, -1.7831) (11.3485, -1.5757) (11.5362, -1.5757) knots 0 0 0 1 2 2 2
  spline S210 degree 2 poles (11.5362, -1.5757) (11.6968, -1.5757) (11.9512, -1.6769) (12.0376, -1.7807) knots 0 0 0 1 2 2 2
  spline S211 degree 2 poles (12.0376, -1.7807) (12.134, -1.8918) (12.2303, -2.1956) (12.2303, -2.4402) knots 0 0 0 1 2 2 2
  line L183 (12.2303, -2.4402) -> (12.2303, -3.937)
  line L184 (12.2303, -3.937) -> (11.509, -3.937)
  line L185 (15.5055, -3.937) -> (15.5055, -2.7884)
  spline S212 degree 2 poles (15.5055, -2.7884) (15.5055, -2.618) (15.4932, -2.3858) (15.4635, -2.3117) knots 0 0 0 1 2 2 2
  spline S213 degree 2 poles (15.4635, -2.3117) (15.4314, -2.2376) (15.303, -2.1709) (15.1869, -2.1709) knots 0 0 0 1 2 2 2
  spline S214 degree 2 poles (15.1869, -2.1709) (15.1054, -2.1709) (14.9473, -2.2426) (14.8534, -2.3093) knots 0 0 0 1 2 2 2
  line L186 (14.8534, -2.3093) -> (14.8534, -3.937)
  line L187 (14.8534, -3.937) -> (14.1322, -3.937)
  line L188 (14.1322, -3.937) -> (14.1322, -2.7884)
  spline S215 degree 2 poles (14.1322, -2.7884) (14.1322, -2.6205) (14.1174, -2.3858) (14.0877, -2.3117) knots 0 0 0 1 2 2 2
  spline S216 degree 2 poles (14.0877, -2.3117) (14.0556, -2.2376) (13.9272, -2.1709) (13.8111, -2.1709) knots 0 0 0 1 2 2 2
  spline S217 degree 2 poles (13.8111, -2.1709) (13.7246, -2.1709) (13.5542, -2.2524) (13.4752, -2.3093) knots 0 0 0 1 2 2 2
  line L189 (13.4752, -2.3093) -> (13.4752, -3.937)
  line L190 (13.4752, -3.937) -> (12.7589, -3.937)
  line L191 (12.7589, -3.937) -> (12.7589, -1.6374)
  line L192 (12.7589, -1.6374) -> (13.4752, -1.6374)
  line L193 (13.4752, -1.6374) -> (13.4752, -1.8918)
  spline S218 degree 2 poles (13.4752, -1.8918) (13.6505, -1.7436) (13.9642, -1.5757) (14.1594, -1.5757) knots 0 0 0 1 2 2 2
  spline S219 degree 2 poles (14.1594, -1.5757) (14.3693, -1.5757) (14.6904, -1.7757) (14.7744, -1.9758) knots 0 0 0 1 2 2 2
  spline S220 degree 2 poles (14.7744, -1.9758) (14.9794, -1.7831) (15.345, -1.5757) (15.5327, -1.5757) knots 0 0 0 1 2 2 2
  spline S221 degree 2 poles (15.5327, -1.5757) (15.6932, -1.5757) (15.9477, -1.6769) (16.0341, -1.7807) knots 0 0 0 1 2 2 2
  spline S222 degree 2 poles (16.0341, -1.7807) (16.1304, -1.8918) (16.2268, -2.1956) (16.2268, -2.4402) knots 0 0 0 1 2 2 2
  line L194 (16.2268, -2.4402) -> (16.2268, -3.937)
  line L195 (16.2268, -3.937) -> (15.5055, -3.937)
  line L196 (-5.3859, -16.8665) -> (-7.6262, -16.8665)
  line L197 (-7.6262, -16.8665) -> (-7.6262, -16.37)
  spline S223 degree 2 poles (-7.6262, -16.37) (-7.3421, -16.1428) (-6.8876, -15.7427) (-6.7172, -15.5624) knots 0 0 0 1 2 2 2
  spline S224 degree 2 poles (-6.7172, -15.5624) (-6.4924, -15.3277) (-6.2924, -14.9696) (-6.2924, -14.7818) knots 0 0 0 1 2 2 2
  spline S225 degree 2 poles (-6.2924, -14.7818) (-6.2924, -14.5694) (-6.5468, -14.3422) (-6.774, -14.3422) knots 0 0 0 1 2 2 2
  spline S226 degree 2 poles (-6.774, -14.3422) (-6.8901, -14.3422) (-7.0976, -14.399) (-7.2038, -14.4434) knots 0 0 0 1 2 2 2
  spline S227 degree 2 poles (-7.2038, -14.4434) (-7.3075, -14.4904) (-7.4557, -14.5892) (-7.4928, -14.6139) knots 0 0 0 1 2 2 2
  line L198 (-7.4928, -14.6139) -> (-7.5521, -14.6139)
  line L199 (-7.5521, -14.6139) -> (-7.5521, -13.9494)
  spline S228 degree 2 poles (-7.5521, -13.9494) (-7.4236, -13.8877) (-6.8753, -13.7592) (-6.6209, -13.7592) knots 0 0 0 1 2 2 2
  spline S229 degree 2 poles (-6.6209, -13.7592) (-6.0775, -13.7592) (-5.5193, -14.2434) (-5.5193, -14.6806) knots 0 0 0 1 2 2 2
  spline S230 degree 2 poles (-5.5193, -14.6806) (-5.5193, -14.9498) (-5.7737, -15.4685) (-6.0676, -15.7649) knots 0 0 0 1 2 2 2
  spline S231 degree 2 poles (-6.0676, -15.7649) (-6.2528, -15.9477) (-6.6011, -16.2317) (-6.6777, -16.291) knots 0 0 0 1 2 2 2
  line L200 (-6.6777, -16.291) -> (-5.3859, -16.291)
  line L201 (-5.3859, -16.291) -> (-5.3859, -16.8665)
  line L202 (-4.2497, -16.8665) -> (-4.9734, -16.8665)
  line L203 (-4.9734, -16.8665) -> (-4.9734, -16.0613)
  line L204 (-4.9734, -16.0613) -> (-4.2497, -16.0613)
  line L205 (-4.2497, -16.0613) -> (-4.2497, -16.8665)
  spline S232 degree 2 poles (-1.4758, -15.8341) (-1.4758, -16.0736) (-1.6389, -16.4787) (-1.7994, -16.6245) knots 0 0 0 1 2 2 2
  spline S233 degree 2 poles (-1.7994, -16.6245) (-1.96, -16.7702) (-2.3996, -16.9307) (-2.7207, -16.9307) knots 0 0 0 1 2 2 2
  spline S234 degree 2 poles (-2.7207, -16.9307) (-3.0616, -16.9283) (-3.5506, -16.8171) (-3.7112, -16.7455) knots 0 0 0 1 2 2 2
  line L206 (-3.7112, -16.7455) -> (-3.7112, -16.0811)
  line L207 (-3.7112, -16.0811) -> (-3.642, -16.0811)
  spline S235 degree 2 poles (-3.642, -16.0811) (-3.5828, -16.1132) (-3.4395, -16.1971) (-3.3234, -16.2416) knots 0 0 0 1 2 2 2
  spline S236 degree 2 poles (-3.3234, -16.2416) (-3.2147, -16.2836) (-2.99, -16.3404) (-2.8541, -16.3404) knots 0 0 0 1 2 2 2
  spline S237 degree 2 poles (-2.8541, -16.3404) (-2.7355, -16.3404) (-2.4589, -16.2811) (-2.3749, -16.2021) knots 0 0 0 1 2 2 2
  spline S238 degree 2 poles (-2.3749, -16.2021) (-2.3132, -16.1403) (-2.244, -15.9897) (-2.244, -15.8637) knots 0 0 0 1 2 2 2
  spline S239 degree 2 poles (-2.244, -15.8637) (-2.244, -15.755) (-2.3329, -15.6019) (-2.4046, -15.5549) knots 0 0 0 1 2 2 2
  spline S240 degree 2 poles (-2.4046, -15.5549) (-2.5083, -15.4858) (-2.8047, -15.4463) (-2.9109, -15.4463) knots 0 0 0 1 2 2 2
  spline S241 degree 2 poles (-2.9109, -15.4463) (-3.0789, -15.4463) (-3.3975, -15.5006) (-3.5136, -15.5302) knots 0 0 0 1 2 2 2
  line L208 (-3.5136, -15.5302) -> (-3.5803, -15.5302)
  line L209 (-3.5803, -15.5302) -> (-3.5803, -13.8185)
  line L210 (-3.5803, -13.8185) -> (-1.5598, -13.8185)
  line L211 (-1.5598, -13.8185) -> (-1.5598, -14.394)
  line L212 (-1.5598, -14.394) -> (-2.8566, -14.394)
  line L213 (-2.8566, -14.394) -> (-2.8566, -14.9004)
  spline S242 degree 2 poles (-2.8566, -14.9004) (-2.7948, -14.8954) (-2.6244, -14.8905) (-2.5775, -14.8905) knots 0 0 0 1 2 2 2
  spline S243 degree 2 poles (-2.5775, -14.8905) (-2.3576, -14.8905) (-1.9871, -14.9794) (-1.8414, -15.0708) knots 0 0 0 1 2 2 2
  spline S244 degree 2 poles (-1.8414, -15.0708) (-1.6685, -15.1844) (-1.4758, -15.5624) (-1.4758, -15.8341) knots 0 0 0 1 2 2 2
  line L214 (2.9603, -16.8665) -> (2.9603, -15.718)
  spline S245 degree 2 poles (2.9603, -15.718) (2.9603, -15.5475) (2.948, -15.3154) (2.9183, -15.2413) knots 0 0 0 1 2 2 2
  spline S246 degree 2 poles (2.9183, -15.2413) (2.8862, -15.1672) (2.7578, -15.1005) (2.6417, -15.1005) knots 0 0 0 1 2 2 2
  spline S247 degree 2 poles (2.6417, -15.1005) (2.5602, -15.1005) (2.4021, -15.1721) (2.3082, -15.2388) knots 0 0 0 1 2 2 2
  line L215 (2.3082, -15.2388) -> (2.3082, -16.8665)
  line L216 (2.3082, -16.8665) -> (1.587, -16.8665)
  line L217 (1.587, -16.8665) -> (1.587, -15.718)
  spline S248 degree 2 poles (1.587, -15.718) (1.587, -15.55) (1.5722, -15.3154) (1.5425, -15.2413) knots 0 0 0 1 2 2 2
  spline S249 degree 2 poles (1.5425, -15.2413) (1.5104, -15.1672) (1.382, -15.1005) (1.2659, -15.1005) knots 0 0 0 1 2 2 2
  spline S250 degree 2 poles (1.2659, -15.1005) (1.1794, -15.1005) (1.009, -15.182) (0.93, -15.2388) knots 0 0 0 1 2 2 2
  line L218 (0.93, -15.2388) -> (0.93, -16.8665)
  line L219 (0.93, -16.8665) -> (0.2137, -16.8665)
  line L220 (0.2137, -16.8665) -> (0.2137, -14.5669)
  line L221 (0.2137, -14.5669) -> (0.93, -14.5669)
  line L222 (0.93, -14.5669) -> (0.93, -14.8213)
  spline S251 degree 2 poles (0.93, -14.8213) (1.1053, -14.6731) (1.419, -14.5052) (1.6142, -14.5052) knots 0 0 0 1 2 2 2
  spline S252 degree 2 poles (1.6142, -14.5052) (1.8241, -14.5052) (2.1452, -14.7053) (2.2292, -14.9053) knots 0 0 0 1 2 2 2
  spline S253 degree 2 poles (2.2292, -14.9053) (2.4342, -14.7127) (2.7998, -14.5052) (2.9875, -14.5052) knots 0 0 0 1 2 2 2
  spline S254 degree 2 poles (2.9875, -14.5052) (3.148, -14.5052) (3.4024, -14.6065) (3.4889, -14.7102) knots 0 0 0 1 2 2 2
  spline S255 degree 2 poles (3.4889, -14.7102) (3.5852, -14.8213) (3.6816, -15.1252) (3.6816, -15.3697) knots 0 0 0 1 2 2 2
  line L223 (3.6816, -15.3697) -> (3.6816, -16.8665)
  line L224 (3.6816, -16.8665) -> (2.9603, -16.8665)
  line L225 (6.9568, -16.8665) -> (6.9568, -15.718)
  spline S256 degree 2 poles (6.9568, -15.718) (6.9568, -15.5475) (6.9445, -15.3154) (6.9148, -15.2413) knots 0 0 0 1 2 2 2
  spline S257 degree 2 poles (6.9148, -15.2413) (6.8827, -15.1672) (6.7543, -15.1005) (6.6382, -15.1005) knots 0 0 0 1 2 2 2
  spline S258 degree 2 poles (6.6382, -15.1005) (6.5567, -15.1005) (6.3986, -15.1721) (6.3047, -15.2388) knots 0 0 0 1 2 2 2
  line L226 (6.3047, -15.2388) -> (6.3047, -16.8665)
  line L227 (6.3047, -16.8665) -> (5.5835, -16.8665)
  line L228 (5.5835, -16.8665) -> (5.5835, -15.718)
  spline S259 degree 2 poles (5.5835, -15.718) (5.5835, -15.55) (5.5687, -15.3154) (5.539, -15.2413) knots 0 0 0 1 2 2 2
  spline S260 degree 2 poles (5.539, -15.2413) (5.5069, -15.1672) (5.3785, -15.1005) (5.2624, -15.1005) knots 0 0 0 1 2 2 2
  spline S261 degree 2 poles (5.2624, -15.1005) (5.1759, -15.1005) (5.0055, -15.182) (4.9264, -15.2388) knots 0 0 0 1 2 2 2
  line L229 (4.9264, -15.2388) -> (4.9264, -16.8665)
  line L230 (4.9264, -16.8665) -> (4.2101, -16.8665)
  line L231 (4.2101, -16.8665) -> (4.2101, -14.5669)
  line L232 (4.2101, -14.5669) -> (4.9264, -14.5669)
  line L233 (4.9264, -14.5669) -> (4.9264, -14.8213)
  spline S262 degree 2 poles (4.9264, -14.8213) (5.1018, -14.6731) (5.4155, -14.5052) (5.6106, -14.5052) knots 0 0 0 1 2 2 2
  spline S263 degree 2 poles (5.6106, -14.5052) (5.8206, -14.5052) (6.1417, -14.7053) (6.2257, -14.9053) knots 0 0 0 1 2 2 2
  spline S264 degree 2 poles (6.2257, -14.9053) (6.4307, -14.7127) (6.7962, -14.5052) (6.984, -14.5052) knots 0 0 0 1 2 2 2
  spline S265 degree 2 poles (6.984, -14.5052) (7.1445, -14.5052) (7.3989, -14.6065) (7.4854, -14.7102) knots 0 0 0 1 2 2 2
  spline S266 degree 2 poles (7.4854, -14.7102) (7.5817, -14.8213) (7.678, -15.1252) (7.678, -15.3697) knots 0 0 0 1 2 2 2
  line L234 (7.678, -15.3697) -> (7.678, -16.8665)
  line L235 (7.678, -16.8665) -> (6.9568, -16.8665)
  dimension "d31" = 15.24
  dimension "d32" = 1.27
  dimension "d33" = 3.937
  constraints: 8 end point, 6 horizontal, 2 parallel, 8 other
  measures "d31" distance from line of L0 point (0, 0)
  measures "d32" distance from line of point (0, 0) L2
  measures "d33" distance from line of L3 point (0, 0)
extrude "Extrusion5" cut sketch "Sketch6" against normal blind 3.175
equation "\"d0\" = outerDiameter"
equation "\"d1\" = depthWiderTopUnit"
equation "\"d3\" = innerDiameter"
equation "\"d4\" = depthLowerUnit"
equation "\"d9\" = screwRadius"
equation "\"d10\" = screwRadius"
equation "\"d23\" = allenKeyHole4_0mm"
equation "\"d24\" = allenKeyHole3_5mm"
equation "\"d25\" = allenKeyHole3_0mm"